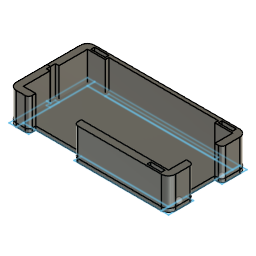
receiver body (Autodesk Fusion 360 design; units mm, degrees)
part number: 2026-04-17-22-42-46-108
Autodesk Fusion 360 part; units mm, degrees
note: some values were not read from the file. Set by a fixed rule: which sketch regions a step uses.
sketch "Sketch1" plane through (0, 0, 0) normal (0, 0, 1) x (1, 0, 0)
  line L0 (-56.8435, 31.9846) -> (24.6565, 31.9846)
  line L1 (24.6565, 31.9846) -> (24.6565, -4.0154)
  line L2 (24.6565, -4.0154) -> (-56.8435, -4.0154)
  line L3 (-56.8435, -4.0154) -> (-56.8435, 31.9846)
  line L4 (-56.8435, -4.0154) -> (-49.8435, -4.0154)
  line L5 (-49.8435, -4.0154) -> (-49.8435, -8.0154)
  line L6 (-49.8435, -8.0154) -> (-56.8435, -8.0154)
  line L7 (-56.8435, -8.0154) -> (-56.8435, -4.0154)
  line L8 (24.6565, -4.0154) -> (-24.3435, -4.0154)
  line L9 (-24.3435, -4.0154) -> (-24.3435, -8.0154)
  line L10 (-24.3435, -8.0154) -> (24.6565, -8.0154)
  line L11 (24.6565, -8.0154) -> (24.6565, -4.0154)
  line L12 (-56.8435, 31.9846) -> (24.6565, 31.9846)
  line L13 (24.6565, 31.9846) -> (24.6565, 35.9846)
  line L14 (24.6565, 35.9846) -> (-56.8435, 35.9846)
  line L15 (-56.8435, 35.9846) -> (-56.8435, 31.9846)
  line L16 (-46.8435, 34) -> (14.6565, 34)
  line L17 (14.6565, 34) -> (14.6565, 31.9846)
  line L18 (14.6565, 31.9846) -> (-46.8435, 31.9846)
  line L19 (-46.8435, 31.9846) -> (-46.8435, 34)
  line L20 (-56.8435, 35.9846) -> (-60.8435, 35.9846)
  line L21 (-60.8435, 35.9846) -> (-60.8435, -8.0154)
  line L22 (-60.8435, -8.0154) -> (-56.8435, -8.0154)
  line L23 (-56.8435, -8.0154) -> (-56.8435, 35.9846)
  line L24 (-56.8435, 15.9846) -> (-58.8435, 15.9846)
  line L25 (-58.8435, 15.9846) -> (-58.8435, 10.9846)
  line L26 (-58.8435, 10.9846) -> (-56.8435, 10.9846)
  line L27 (-56.8435, 10.9846) -> (-56.8435, 15.9846)
  line L28 (-60.8435, 13.2091) -> (-58.8435, 13.2091)
  line L29 (-58.8435, 13.2091) -> (-58.8435, 13.1879)
  line L30 (-58.8435, 13.1879) -> (-60.8435, 13.1879)
  line L31 (-60.8435, 13.1879) -> (-60.8435, 13.2091)
  line L32 (24.6565, 25.9846) -> (24.6565, 35.9846)
  line L33 (24.6565, 1.9846) -> (24.6565, -8.0154)
  line L34 (24.6565, -8.0154) -> (28.6565, -8.0154)
  line L35 (28.6565, -8.0154) -> (28.6565, 5.9846)
  line L36 (28.6565, 5.9846) -> (24.6565, 5.9846)
  line L37 (24.6565, 5.9846) -> (24.6565, -8.0154)
  line L38 (24.6565, 35.9846) -> (28.6565, 35.9846)
  line L39 (28.6565, 35.9846) -> (28.6565, 21.9846)
  line L40 (28.6565, 21.9846) -> (24.6565, 21.9846)
  line L41 (24.6565, 21.9846) -> (24.6565, 35.9846)
  dimension "d1" = 81.5
  dimension "d2" = 36
  dimension "d3" = 7
  dimension "d4" = 4
  dimension "d5" = 49
  dimension "d6" = 4
  dimension "d7" = 4
  dimension "d8" = 10
  dimension "d9" = 10
  dimension "d10" = 4
  dimension "d11" = 44
  dimension "d12" = 2
  dimension "d13" = 5
  dimension "d15" = 19
  dimension "d16" = 2
  dimension "d18" = 10
  dimension "d20" = 10
  dimension "d23" = 4
  dimension "d24" = 14
  dimension "d25" = 4
  dimension "d26" = 14
  constraint horizontal L0
  constraint vertical L1
  constraint horizontal L2
  constraint vertical L3
  constraint horizontal L4
  constraint vertical L5
  constraint horizontal L6
  constraint vertical L7
  constraint horizontal L8
  constraint vertical L9
  constraint horizontal L10
  constraint vertical L11
  constraint horizontal L12
  constraint vertical L13
  constraint horizontal L14
  constraint vertical L15
  constraint horizontal L16
  constraint vertical L17
  constraint horizontal L18
  constraint vertical L19
  constraint coincident L12 L17.end
  constraint horizontal L20
  constraint vertical L21
  constraint horizontal L22
  constraint vertical L23
  constraint horizontal L24
  constraint vertical L25
  constraint horizontal L26
  constraint vertical L27
  constraint horizontal L28
  constraint vertical L29
  constraint horizontal L30
  constraint vertical L31
  constraint coincident L25 L29.end
  constraint coincident L21 L28.start
  constraint vertical L32
  constraint vertical L33
  constraint horizontal L34
  constraint vertical L35
  constraint horizontal L36
  constraint vertical L37
  constraint horizontal L38
  constraint vertical L39
  constraint horizontal L40
  constraint vertical L41
  measures "d1" distance of L0.start L0.end
  measures "d2" distance of L0.start L2.end
  measures "d3" distance of L2.end L4.end
  measures "d4" distance of L2.end L6.end
  measures "d5" distance of L1.end L8.end
  measures "d6" distance of L1.end L10.end
  measures "d7" distance of L0.start L14.end
  measures "d8" distance of L15 L19
  measures "d9" distance of L13 L17
  measures "d10" distance of L14.end L20.end
  measures "d11" distance of L14.end L6.end
  measures "d12" distance of L24.start L24.end
  measures "d13" distance of L24.start L26.end
  measures "d15" distance of L22 L26
  measures "d16" distance of L21 L25
  measures "d18" distance of L13.end L32.start
  measures "d20" distance of L10.end L33.start
  measures "d23" distance of L10.end L34.end
  measures "d24" distance of L10.end L36.end
  measures "d25" distance of L13.end L38.end
  measures "d26" distance of L13.end L40.end
extrude "Extrude1" add sketch "Sketch1" along normal blind 2 makes body 1
extrude "Extrude2" add sketch "Sketch1" along normal blind 17.8 separate body contours L0 L12 L13 L14 L15 L16 L17 L19 L23 L32 L41 | L3 L15 L20 L21 L23 L24 L25 L28 | L3 L7 L21 L22 L23 L25 L26 L30 | L1 L13 L32 L38 L39 L40 L41 | L2 L4 L5 L6 L7 L23 | L2 L8 L9 L10 L11 L33 L37 | L1 L11 L33 L34 L35 L36 L37 makes body 2 at (-1.1768, 35.9846, 5.9333) makes body 3 at (10.9898, -8.0154, 11.8667) makes body 4 at (-60.8435, 6.1202, 5.9333)
fillet "Fillet1" radius 4 4 edges at (28.6565, 35.9846, 8.9) (-60.8435, 35.9846, 8.9) (28.6565, -8.0154, 8.9) (-60.8435, -8.0154, 8.9) on bodies 2 3 4
fillet "Fillet2" radius 4 4 edges at (28.6565, -8.0154, 1) (28.6565, 35.9846, 1) (-60.8435, -8.0154, 1) (-60.8435, 35.9846, 1) on bodies 1
fillet "Fillet3" radius 2 4 edges at (28.6565, 21.9846, 8.9) (-24.3435, -8.0154, 8.9) (28.6565, 5.9846, 8.9) (-49.8435, -8.0154, 8.9) on bodies 2 3 4
fillet "Fillet4" radius 2 2 edges at (-24.3435, -8.0154, 1) (-49.8435, -8.0154, 1) on bodies 1
fillet "Fillet5" radius 2 2 edges at (28.6565, 21.9846, 1) (28.6565, 5.9846, 1) on bodies 1
sketch "Sketch2" plane through (0, 0, 17.8) normal (0, 0, 1) x (-1, 0, 0)
  arc A0 (-26.6565, -21.9846) -> (-28.6565, -23.9846) centre (-26.6565, -23.9846) ccw
  line L0 (-28.6565, -23.9846) -> (-28.6565, -31.9846)
  arc A1 (-28.6565, -31.9846) -> (-24.6565, -35.9846) centre (-24.6565, -31.9846) ccw
  line L1 (-24.6565, -35.9846) -> (56.8435, -35.9846)
  arc A2 (56.8435, -35.9846) -> (60.8435, -31.9846) centre (56.8435, -31.9846) ccw
  line L2 (60.8435, -31.9846) -> (60.8435, -13.2091)
  line L3 (60.8435, -13.2091) -> (58.8435, -13.2091)
  line L4 (58.8435, -13.2091) -> (58.8435, -15.9846)
  line L5 (58.8435, -15.9846) -> (56.8435, -15.9846)
  line L6 (56.8435, -15.9846) -> (56.8435, -31.9846)
  line L7 (56.8435, -31.9846) -> (46.8435, -31.9846)
  line L8 (46.8435, -31.9846) -> (46.8435, -34)
  line L9 (46.8435, -34) -> (-14.6565, -34)
  line L10 (-14.6565, -34) -> (-14.6565, -31.9846)
  line L11 (-14.6565, -31.9846) -> (-24.6565, -31.9846)
  line L12 (-24.6565, -31.9846) -> (-24.6565, -21.9846)
  line L13 (-24.6565, -21.9846) -> (-26.6565, -21.9846)
  line L14 (-23.6565, -32.9846) -> (-15.6565, -32.9846)
  line L15 (-15.6565, -32.9846) -> (-15.6565, -34.9846)
  line L16 (-15.6565, -34.9846) -> (-23.6565, -34.9846)
  line L17 (-23.6565, -34.9846) -> (-23.6565, -32.9846)
  line L18 (56.8435, -31.9846) -> (-24.6565, -31.9846)
  line L19 (-28.6565, -35.9846) -> (-28.6565, -21.9846)
  line L20 (-23.6565, 7.0154) -> (-15.6565, 7.0154)
  line L21 (-15.6565, 7.0154) -> (-15.6565, 5.0154)
  line L22 (-15.6565, 5.0154) -> (-23.6565, 5.0154)
  line L23 (-23.6565, 5.0154) -> (-23.6565, 7.0154)
  line L24 (47.8435, -32.9846) -> (55.8435, -32.9846)
  line L25 (55.8435, -32.9846) -> (55.8435, -34.9846)
  line L26 (55.8435, -34.9846) -> (47.8435, -34.9846)
  line L27 (47.8435, -34.9846) -> (47.8435, -32.9846)
  line L28 (-28.6565, 8.0154) -> (-28.6565, -5.9846)
  line L29 (24.3435, 8.0154) -> (-24.6565, 8.0154)
  line L30 (60.8435, -35.9846) -> (60.8435, 8.0154)
  line L31 (-24.6565, -35.9846) -> (56.8435, -35.9846)
  line L32 (56.8435, -31.9846) -> (-24.6565, -31.9846)
  dimension "d39" = 8
  dimension "d40" = 2
  dimension "d41" = 1
  dimension "d42" = 5
  dimension "d43" = 8
  dimension "d44" = 2
  dimension "d45" = 8
  dimension "d46" = 2
  dimension "d47" = 5
  dimension "d48" = 1
  dimension "d49" = 5
  dimension "d51" = 1
  constraint horizontal L14
  constraint vertical L15
  constraint horizontal L16
  constraint vertical L17
  constraint horizontal L20
  constraint vertical L21
  constraint horizontal L22
  constraint vertical L23
  constraint horizontal L24
  constraint vertical L25
  constraint horizontal L26
  constraint vertical L27
  measures "d39" distance of L14.start L14.end
  measures "d40" distance of L14.start L16.end
  measures "d41" distance of L14 L18
  measures "d42" distance of L17 L19
  measures "d43" distance of L20.start L20.end
  measures "d44" distance of L20.start L22.end
  measures "d45" distance of L24.start L24.end
  measures "d46" distance of L24.start L26.end
  measures "d47" distance of L23 L28
  measures "d48" distance of L20 L29
  measures "d49" distance of L25 L30
  measures "d51" distance of L24 L32
extrude "Extrude4" cut sketch "Sketch2" against normal blind 8 contours L14 L15 L16 L17 | L20 L21 L22 L23 | L24 L25 L26 L27 bodies 2 3
extrude "Extrude3" [suppressed]
delete_face "DeleteFace1" [suppressed]
delete_face "DeleteFace2" [suppressed]
delete_face "DeleteFace3" [suppressed]
